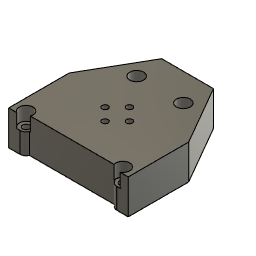
Gripper_Mount_v3 (Autodesk Fusion 360 design; units mm, degrees)
Autodesk Fusion 360 part; units mm, degrees
sketch "Sketch1" plane through (0, 0, 0) normal (0, 1, 0) x (1, 0, 0)
  line L0 (-7, 0) -> (-6, 0)
  line L1 (-24.7504, 0) -> (24.7504, 0)
  line L2 (-28, -2.2) -> (-34.6, -2.2)
  line L3 (28, -2.2) -> (34.6, -2.2)
  line L4 (-34.6, -2.2) -> (-34.6, 32.8)
  line L5 (-13.5, 50.8) -> (13.5, 50.8) construction
  line L6 (34.6, 32.8) -> (34.6, -2.2)
  line L7 (0, 0) -> (0, 50.8) construction
  arc A0 (-28, -2.2) -> (-24.7504, 0) centre (-28, 1.3) ccw
  arc A1 (24.7504, 0) -> (28, -2.2) centre (28, 1.3) ccw
  circle A2 centre (-13.5, 50.8) radius 2
  circle A3 centre (13.5, 50.8) radius 2
  circle A4 centre (-28, 1.3) radius 2
  circle A5 centre (-28, 1.3) radius 4
  circle A6 centre (28, 1.3) radius 4
  circle A7 centre (28, 1.3) radius 2
  circle A8 centre (-13.5, 50.8) radius 4
  circle A9 centre (13.5, 50.8) radius 4
  line L8 (0, 66.7482) -> (0, 50.8) construction
  line L9 (-15, 66.7482) -> (-34.6, 32.8)
  line L10 (15, 66.7482) -> (34.6, 32.8)
  line L11 (-15, 66.7482) -> (15, 66.7482)
  line L12 (0, 33.1421) -> (-7.0711, 26.0711) construction
  line L13 (-7.0711, 26.0711) -> (0, 19) construction
  line L14 (0, 33.1421) -> (-0.7721, 33.9142) construction
  line L15 (-0.7721, 33.9142) -> (7.0711, 26.0711) construction
  line L16 (7.0711, 26.0711) -> (0, 19) construction
  circle A10 centre (0, 33.1421) radius 1.75
  circle A11 centre (-7.0711, 26.0711) radius 1.75
  circle A12 centre (0, 19) radius 1.75
  circle A13 centre (7.0711, 26.0711) radius 1.75
  circle A14 centre (0, 33.1421) radius 3.5
  circle A15 centre (-7.0711, 26.0711) radius 3.5
  circle A16 centre (0, 19) radius 3.5
  circle A17 centre (7.0711, 26.0711) radius 3.5
  point P0 (0, 44.2)
  dimension "d10" = 6.6
  dimension "d11" = 6.6
  dimension "d12" = 35
  dimension "d13" = 35
  dimension "d14" = 49.5
  dimension "d15" = 27
  dimension "d18" = 1.3
  dimension "d19" = 1.3
  dimension "d20" = 3.5
  dimension "d21" = 3.5
  dimension "d35" = 8
  dimension "d36" = 8
  dimension "d37" = 8
  dimension "d38" = 8
  dimension "d39" = 4
  dimension "d40" = 4
  dimension "d41" = 4
  dimension "d42" = 4
  dimension "d43" = 56
  dimension "d52" = 150
  dimension "d53" = 150
  dimension "d70" = 30
  dimension "d71" = 10
  dimension "d72" = 3.5
  dimension "d73" = 3.5
  dimension "d74" = 3.5
  dimension "d75" = 3.5
  dimension "d76" = 7
  dimension "d77" = 7
  dimension "d78" = 7
  dimension "d79" = 7
  dimension "d84" = 19
  constraint horizontal L0
  constraint horizontal L1
  constraint tangent L2 A0
  constraint tangent L3 A1
  constraint perpendicular L2 L4
  constraint vertical L6
  constraint coincident L7.start origin
  constraint midpoint L5 L7.end
  constraint vertical L7
  constraint horizontal L5
  constraint coincident L7.start L1
  constraint vertical L4
  constraint horizontal L3
  constraint coincident L7 P0
  constraint coincident L5.start A2.centre
  constraint concentric A2 A8
  constraint coincident L5.end A3.centre
  constraint concentric A3 A9
  constraint concentric A0 A4
  constraint concentric A4 A5
  constraint concentric A1 A6
  constraint concentric A6 A7
  constraint midpoint L7.start L1
  constraint midpoint L8.start L11
  constraint vertical L8
  constraint coincident L7 L12.start
  constraint coincident L7 L13.end
  constraint perpendicular L12 L13
  constraint perpendicular L12 L14
  constraint perpendicular L12 L15
  constraint perpendicular L13 L16
  constraint coincident L12.start L14.start
  constraint coincident L12.end L13.start
  constraint coincident L13.end L16.end
  constraint coincident L15.end L16.start
  constraint concentric A10 A14
  constraint concentric A11 A15
  constraint concentric A12 A16
  constraint concentric A13 A17
  measures "d10" distance of L2.start L2.end
  measures "d11" distance of L3.start L3.end
  measures "d12" distance of L2.end L4.end
  measures "d13" distance of L3.end L6.start
  measures "d14" distance of A1.centre L5
  measures "d15" distance of L5.start L5.end
  measures "d18" distance of A0.centre L1
  measures "d19" distance of A1.centre L1
  measures "d20" radius of A0
  measures "d21" radius of A1
  measures "d35" diameter of A8
  measures "d36" diameter of A9
  measures "d37" diameter of A5
  measures "d38" diameter of A6
  measures "d39" diameter of A2
  measures "d40" diameter of A3
  measures "d41" diameter of A4
  measures "d42" diameter of A7
  measures "d43" distance of A0.centre A1.centre
  measures "d52" angle of L4 L9
  measures "d53" angle of L6 L10
  measures "d70" distance of L10.start L9.start
  measures "d71" distance of L12.start L12.end
  measures "d72" diameter of A10
  measures "d73" diameter of A11
  measures "d74" diameter of A13
  measures "d75" diameter of A12
  measures "d76" diameter of A14
  measures "d77" diameter of A15
  measures "d78" diameter of A17
  measures "d79" diameter of A16
  measures "d84" distance of L1 L13.end
extrude "Extrude1" add sketch "Sketch1" along normal blind 20 contours L0 L1 L2 L3 L4 L6 A5 A6 L9 L10 L11 | L1 L2 A0 A5 | L1 L3 A1 A6 | A2 | A3 | A4 | A7 | A8 | A9 | A10 | A11 | A12 | A13 | A14 | A15 | A16 | A17 picked at (-28.8891, -1.6539) picked at (28.8891, -1.6539)
extrude "Extrude2" cut sketch "Sketch1" along normal blind 20 contours A2 | A3 | A4 | A7
extrude "Extrude3" cut sketch "Sketch1" against normal blind 8 from surface at 20 contours L1 L2 A0 A5 | L1 L3 A1 A6 | A8 | A9 picked at (-28.8891, -1.6539) picked at (28.8891, -1.6539)
extrude "Extrude7" cut sketch "Sketch1" along normal blind 20 contours A10 | A11 | A12 | A13
extrude "Extrude8" cut sketch "Sketch1" along normal blind 3.5 contours A14 | A15 | A16 | A17
